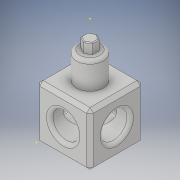
# Autodesk Inventor part: orthographic3
Saved by Autodesk Inventor 2017 (Build 210142000, 142)
## iProperties
Created: 2018-11-30
Part Number: orthographic3
Material: Generic
Document SubType Name: Modeling
Designer: qthuynh
Density: 1 g/cm^3
Appearance: Default
Author: qthuynh
Autodesk Inventor part; units mm, degrees
ref_plane "YZ Plane" through (0, 0, 0) normal (1, 0, 0) x (0, 1, 0)
ref_plane "XZ Plane" through (0, 0, 0) normal (0, 1, 0) x (-1, 0, 0)
ref_plane "XY Plane" through (0, 0, 0) normal (0, 0, 1) x (1, 0, 0)
sketch "Sketch1" plane through (0, 0, 0) normal (0, 0, 1) x (1, 0, 0)
  line L0 (0, 0) -> (50.8, 0)
  line L1 (50.8, 0) -> (50.8, 50.8)
  line L2 (50.8, 50.8) -> (0, 50.8)
  line L3 (0, 50.8) -> (0, 0)
  dimension "d0" = 50.8
  dimension "d1" = 50.8
  constraints: 8 end point, 2 parallel, 1 horizontal, 1 perpendicular
  measures "d0" distance of L2.end L1.end
  measures "d1" distance of L1.end L0.end
extrude "Extrusion1" add sketch "Sketch1" along normal blind 50.8
sketch "Sketch2" plane through (0, 0, 50.8) normal (0, 0, 1) x (1, 0, 0)
  point P0 (0, 0)
sketch "Sketch3" plane through (0, 0, 50.8) normal (0, 0, 1) x (1, 0, 0)
  circle A0 centre (25.4, 25.4) radius 12.7
  line L0 (0, 50.8) -> (0, 0) projected
  line L1 (50.8, 50.8) -> (0, 50.8) projected
  dimension "d4" = 25.4
  dimension "d5" = 25.4
  dimension "d6" = 25.4
  constraints: 1 centre point
  measures "d4" diameter of A0
  measures "d5" distance from line of L0 A0.centre
  measures "d6" distance from line of L1 A0.centre
extrude "Extrusion2" cut sketch "Sketch3" against normal blind 50.8
sketch "Sketch4" plane through (50.8, 0, 0) normal (1, 0, 0) x (0, 0, -1)
  circle A0 centre (-25.4, 25.4) radius 12.7
  line L0 (-50.8, 0) -> (-50.8, 50.8) projected
  line L1 (0, 0) -> (0, 50.8) projected
  line L2 (0, 0) -> (-50.8, 0) projected
  dimension "d9" = 25.4
  dimension "d10" = 25.4
  dimension "d11" = 25.4
  dimension "d12" = 25.4
  constraints: 1 centre point
  measures "d9" diameter of A0
  measures "d10" distance from line of L0 A0.centre
  measures "d11" distance from line of L1 A0.centre
  measures "d12" distance from line of L2 A0.centre
extrude "Extrusion3" cut sketch "Sketch4" against normal blind 50.8
chamfer "Chamfer1" distance 3.175 angle 45 12 edges at (25.4, 50.8, 50.8) (0, 50.8, 25.4) (25.4, 50.8, 0) (50.8, 50.8, 25.4) (50.8, 25.4, 50.8) (50.8, 25.4, 0) (50.8, 0, 25.4) (25.4, 0, 0) (25.4, 0, 50.8) (0, 25.4, 50.8) (0, 0, 25.4) (0, 25.4, 0)
fillet "Fillet1" radius 3.175 4 edges at (12.7, 25.4, 50.8) (50.8, 25.4, 38.1) (12.7, 25.4, 0) (0, 25.4, 38.1)
sketch "Sketch5" plane through (3.175, 50.8, 3.175) normal (0, 1, 0) x (1, 0, 0)
  line L0 (22.225, -22.225) -> (9.525, -34.925) projected
  circle A0 centre (22.225, -22.225) radius 12.7
  point P0 (-3.175, 3.175)
  dimension "d19" = 25.4
  constraints: 1 centre point
  measures "d19" diameter of A0
extrude "Extrusion4" add sketch "Sketch5" along normal blind 25.4
sketch "Sketch6" plane through (25.4, 76.2, 25.4) normal (0, 1, 0) x (1, 0, 0)
  point P0 (-25.4, 25.4)
fillet "Fillet2" radius 3.175 1 edges at (12.7, 76.2, 25.4)
sketch "Sketch9" plane through (25.4, 76.2, 25.4) normal (0, 1, 0) x (1, 0, 0)
  line L0 (0, 0) -> (12.7, 12.7) projected
  circle A0 centre (0, 0) radius 6.35
  line L1 (0, 6.35) -> (5.4993, 3.175)
  line L2 (5.4993, 3.175) -> (5.4993, -3.175)
  line L3 (5.4993, -3.175) -> (0, -6.35)
  line L4 (0, -6.35) -> (-5.4993, -3.175)
  line L5 (-5.4993, -3.175) -> (-5.4993, 3.175)
  line L6 (-5.4993, 3.175) -> (0, 6.35)
  point P0 (-25.4, 25.4)
  dimension "d25" = 12.7
  constraints: 12 end point, 1 coincident, 1 vertical alignment, 15 other
extrude "Extrusion6" add sketch "Sketch9" along normal blind 9.652 contours L1 L2 L3 L4 L5 L6
chamfer "Chamfer2" distance 0.7937 angle 45 6 edges at (22.6504, 85.852, 30.1625) (28.1496, 85.852, 30.1625) (30.8993, 85.852, 25.4) (22.6504, 85.852, 20.6375) (28.1496, 85.852, 20.6375) (19.9007, 85.852, 25.4)
body "Solid1"
